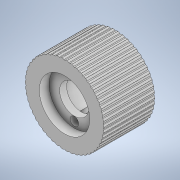
# Autodesk Inventor part: runner
Saved by Autodesk Inventor 2022 (Build 260153000, 153)
## iProperties
Created: 2023-12-11
Part Number: runner
Material: Generisch
Document SubType Name: Modeling
Designer: Marc Panse
Density: 1 g/cm^3
Appearance: Vorgabe
Author: Marc Panse
## iProperties of the stored document runner_3D-Druck.ipt
Created: 2023-12-11
Part Number: runner_3D-Druck
Material: Generisch
Document SubType Name: Modeling
Designer: Marc Panse
Density: 1 g/cm^3
Appearance: Vorgabe
Author: Marc Panse
Autodesk Inventor part; units mm, degrees
ref_plane "YZ Plane" through (0, 0, 0) normal (1, 0, 0) x (0, 1, 0)
ref_plane "XZ Plane" through (0, 0, 0) normal (0, 1, 0) x (-1, 0, 0)
ref_plane "XY Plane" through (0, 0, 0) normal (0, 0, 1) x (1, 0, 0)
sketch "Skizze1" plane through (0, 0, 0) normal (0, 0, 1) x (1, 0, 0)
  circle A0 centre (0, 0) radius 24
  circle A1 centre (0, 0) radius 28.2
  dimension "d0" = 48
  dimension "d1" = 56.4
  constraints: 2 centre point, 2 coincident
  measures "d0" diameter of A0
  measures "d1" diameter of A1
extrude "Extrusion1" add sketch "Skizze1" along normal blind 14
sketch "Skizze2" plane through (0, 0, 0) normal (0, 0, -1) x (-1, 0, 0)
  circle A0 centre (0, 0) radius 24.95
  dimension "d4" = 49.9
  constraints: 1 centre point, 1 coincident
  measures "d4" diameter of A0
extrude "Extrusion2" cut sketch "Skizze2" against normal blind 0.9
sketch "Skizze3" plane through (0, 0, 14) normal (0, 0, 1) x (1, 0, 0)
  circle A0 centre (0, 0) radius 28.2 projected
  circle A1 centre (0, 0) radius 24 projected
  circle A2 centre (0, 0) radius 11.5
  dimension "d7" = 23
  constraints: 1 centre point, 1 coincident
  measures "d7" diameter of A2
extrude "Extrusion3" add sketch "Skizze3" along normal blind 7.4 contours A0 | A1
sketch "Skizze4" plane through (0, 0, 21.4) normal (0, 0, 1) x (1, 0, 0)
  circle A0 centre (0, 0) radius 10.5
  circle A1 centre (0, 0) radius 28.2 projected
  circle A2 centre (0, 0) radius 11.5 projected
  dimension "d10" = 21
  constraints: 1 centre point, 1 coincident
  measures "d10" diameter of A0
extrude "Extrusion4" add sketch "Skizze4" against normal blind 5 contours A2
sketch "Skizze5" plane through (0, 0, 21.4) normal (0, 0, 1) x (1, 0, 0)
  circle A0 centre (0, 0) radius 29.0057
  circle A1 centre (0, 0) radius 10.8
  circle A2 centre (0, 0) radius 18
  circle A3 centre (0, 0) radius 10.5 projected
  circle A4 centre (0, 0) radius 28.2 projected
  dimension "d13" = 36
  constraints: 3 centre point, 3 coincident
  measures "d13" diameter of A2
extrude "Extrusion5" add sketch "Skizze5" along normal blind 7 contours A4
sketch "Skizze6" plane through (0, 0, 14) normal (0, 0, -1) x (-1, 0, 0)
  circle A0 centre (0, 0) radius 11.5 projected
  circle A1 centre (0, 0) radius 24 projected
extrude "Extrusion6" add sketch "Skizze6" along normal blind 8
sketch "Skizze7" plane through (0, 0, 0) normal (0, 0, -1) x (-1, 0, 0)
  point P0 (0, 0)
sketch "Skizze8" plane through (0, 0, 0) normal (0, 0, -1) x (-1, 0, 0)
  circle A0 centre (0, 0) radius 24.95 projected
  circle A1 centre (0, 0) radius 28.2 projected
extrude "Extrusion7" add sketch "Skizze8" along normal blind 8
sketch "Skizze9" plane through (0, 0, 0.9) normal (0, 0, -1) x (-1, 0, 0)
  circle A0 centre (0, 0) radius 24 projected
  circle A1 centre (0, 0) radius 24.95 projected
extrude "Extrusion8" add sketch "Skizze9" along normal blind 8
sketch "Skizze10" plane through (0, 0, 21.4) normal (0, 0, 1) x (1, 0, 0)
  circle A0 centre (0, 0) radius 13.758
  circle A1 centre (0, -13.758) radius 3.05
  dimension "d22" = 27.516
  dimension "d23" = 6.1
  constraints: 1 centre point, 1 coincident, 1 vertical alignment, 2 other
  measures "d23" diameter of A1
extrude "Extrusion9" cut sketch "Skizze10" against normal blind 14 contours A1 A0 | A0 A1 picked at (0, -12.7162) picked at (-0.0564, -14.748)
sketch "Skizze11" plane through (0, 0, -8) normal (0, 0, -1) x (-1, 0, 0)
  circle A0 centre (0, 0) radius 28.2 projected
  circle A1 centre (0, -28.2) radius 0.6087
  constraints: 1 centre point, 1 vertical alignment, 1 other
extrude "Extrusion10" cut sketch "Skizze11" against normal blind 57 contours A1 A0 | A0 A1 picked at (-0.0243, -27.9981) picked at (0.0235, -28.4011)
fillet "Rundung1" radius 2 4 edges at (-0.6086, -28.1934, -4) (-0.6086, -28.1934, 14.2) (0.6086, -28.1934, -4) (0.6086, -28.1934, 14.2)
pattern_circular "Runde Anordnung1" count 50 over 360 about axis through (0, 0, -10) along (0, 0, 1) of "Extrusion10", "Rundung1"
